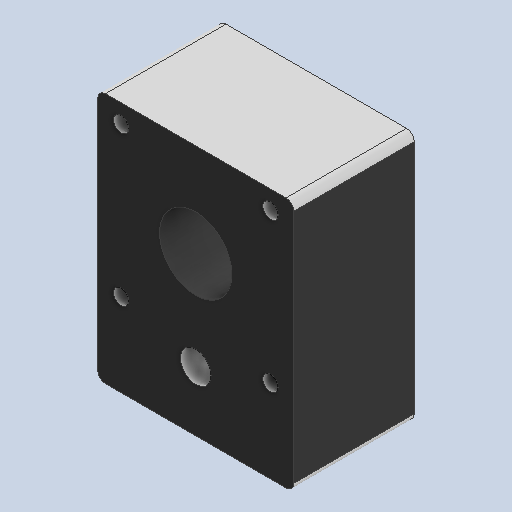
# Autodesk Inventor part: Motor Brace
Saved by Autodesk Inventor 2025.1 (Build 291241020, 241B)
## iProperties
Created: 2025-01-21
Part Number: Motor Brace
Material: Generic
Document SubType Name: Modeling
Designer: Sven
Density: 1 g/cm^3
Appearance: Default
Author: Sven
Autodesk Inventor part; units mm, degrees
ref_plane "YZ Plane" through (0, 0, 0) normal (1, 0, 0) x (0, 1, 0)
ref_plane "XZ Plane" through (0, 0, 0) normal (0, 1, 0) x (-1, 0, 0)
ref_plane "XY Plane" through (0, 0, 0) normal (0, 0, 1) x (1, 0, 0)
sketch "Sketch1" plane through (0, 0, 0) normal (0, 0, 1) x (1, 0, 0)
  line L0 (-20.32, 26.67) -> (20.32, 26.67)
  line L1 (20.32, 26.67) -> (20.32, -26.67)
  line L2 (20.32, -26.67) -> (-20.32, -26.67)
  line L3 (-20.32, -26.67) -> (-20.32, 26.67)
  point P0 (0, 0)
  point P1 (20.32, 0)
  point P2 (0, 26.67)
  dimension "d0" = 40.64
  dimension "d1" = 53.34
  constraints: 8 end point, 2 midpoint, 2 parallel, 1 horizontal, 1 horizontal alignment, 1 perpendicular, 1 vertical alignment
  measures "d0" distance of L0.start L0.end
  measures "d1" distance of L0.end L1.end
extrude "Extrusion1" add sketch "Sketch1" along normal blind 25
sketch "Sketch2" plane through (0, 0, 25) normal (0, 0, 1) x (1, 0, 0)
  circle A0 centre (0, 6.0325) radius 7.5
  line L0 (20.32, 26.67) -> (-20.32, 26.67) projected
  circle A1 centre (0, -14.2875) radius 3.175
  line L1 (0, 6.0325) -> (44.8131, 6.0325) construction
  line L2 (0, 6.0325) -> (0, 52.3228) construction
  circle A2 centre (15.5, 21.5325) radius 1.5875
  circle A3 centre (-15.5, 21.5325) radius 1.5875
  circle A4 centre (15.5, -9.4675) radius 1.5875
  circle A5 centre (-15.5, -9.4675) radius 1.5875
  point P0 (0, 0)
  dimension "d4" = 20.6375
  dimension "d5" = 15
  dimension "d8" = 6.35
  dimension "d9" = 20.32
  dimension "d11" = 3.175
  dimension "d12" = 15.5
  dimension "d13" = 15.5
  constraints: 6 centre point, 4 end point, 3 symmetric about line, 2 vertical alignment, 1 horizontal, 1 vertical, 3 other
  measures "d4" distance from line of L0 L1.start
  measures "d5" diameter of A0
  measures "d8" diameter of A1
  measures "d9" distance of A1.centre L1.start
  measures "d11" diameter of A2
  measures "d12" distance from line of L1 A2.centre
  measures "d13" distance from line of L2 A2.centre
extrude "Extrusion2" cut sketch "Sketch2" against normal up to surface (25 mm away)
sketch "Sketch3" plane through (-20.32, 26.67, 0) normal (0, 1, 0) x (1, 0, 0)
  line L0 (0, 0) -> (0, -25) projected
  line L1 (0, -25) -> (40.64, -25) projected
  line L2 (0, 0) -> (40.64, 0)
  line L3 (40.64, 0) -> (40.64, -25)
  line L4 (40.64, -25) -> (0, -25)
  line L5 (0, -25) -> (0, 0)
  point P0 (20.32, 0)
  constraints: 8 end point, 2 parallel, 1 horizontal, 1 perpendicular
extrude "Extrusion3" cut sketch "Sketch3" against normal blind 1.27
fillet "Fillet1" radius 1.6002 4 edges at (20.32, 25.4, 12.5) (-20.32, 25.4, 12.5) (20.32, -26.67, 12.5) (-20.32, -26.67, 12.5)
body "Solid1"
